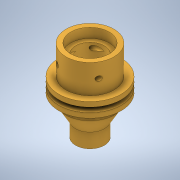
# Autodesk Inventor part: inner element
Saved by Autodesk Inventor 2021 (Build 250183000, 183)
## iProperties
Created: 2021-07-21
Part Number: inner element
Material: Brass, Soft Yellow
Document SubType Name: Modeling
Designer: samlo
Density: 8.47 g/cm^3
Appearance: Brass - Satin
Author: samlo
Autodesk Inventor part; units mm, degrees
ref_plane "YZ Plane" through (0, 0, 0) normal (1, 0, 0) x (0, 1, 0)
ref_plane "XZ Plane" through (0, 0, 0) normal (0, 1, 0) x (-1, 0, 0)
sketch "Sketch1" plane through (0, 0, 0) normal (0, 0, 1) x (1, 0, 0)
  line L0 (2, 0) -> (2, 7)
  line L1 (2, 7) -> (3, 8.7321)
  line L2 (3, 8.7321) -> (3, 15)
  line L3 (3, 15) -> (4, 15)
  line L4 (4, 15) -> (4, 17)
  line L5 (4, 17) -> (5, 17)
  line L6 (5, 17) -> (5, 11)
  line L7 (5, 11) -> (6.5, 11)
  line L8 (6.5, 11) -> (6.5, 10)
  line L9 (6.5, 10) -> (5, 10)
  line L10 (5, 10) -> (5, 9)
  line L11 (5, 9) -> (6.5, 9)
  line L12 (6.5, 9) -> (6.5, 8)
  line L13 (6.5, 8) -> (5, 8)
  line L14 (5, 8) -> (5, 6.4641)
  line L15 (5, 6.4641) -> (3, 3)
  line L16 (3, 3) -> (3, 0)
  line L17 (3, 0) -> (2, 0)
  line L18 (0, -3.4) -> (0, 20.4) projected
  point P0 (0, 0)
  dimension "d0" = 7
  dimension "d1" = 17
  dimension "d2" = 2
  dimension "d3" = 3
  dimension "d4" = 1
  dimension "d5" = 1
  dimension "d6" = 1
  dimension "d7" = 2
  dimension "d8" = 11
  dimension "d9" = 1.5
  dimension "d10" = 5
  dimension "d11" = 60
  dimension "d13" = 4
  dimension "d14" = 3
  dimension "d48" = 4
  constraints: 36 end point, 10 perpendicular, 8 point on line, 2 parallel, 1 vertical
  measures "d0" distance of L0.start L0.end
  measures "d1" vertical distance of L4.end L0.start
  measures "d2" distance of L0.start point (0, 0)
  measures "d3" distance of L16.end point (0, 0)
  measures "d4" distance of L11.end L12.end
  measures "d5" distance of L7.end L8.end
  measures "d6" distance of L9.end L10.end
  measures "d7" distance of L3.end L4.end
  measures "d8" vertical distance of L7.end point (0, 0)
  measures "d9" distance of L12.end L13.end
  measures "d10" horizontal distance of L14.end point (0, 0)
  measures "d11" angle of L17 L1
  measures "d13" distance from line of L4 point (0, 0)
  measures "d14" distance of L15.end L16.end
  measures "d48" distance of L14.end L15.end
revolve "Revolution1" add sketch "Sketch1" angle 360 about axis through (0, -10, 0) along (0, 1, 0)
sketch "Sketch2" plane through (0, 0, 0) normal (1, 0, 0) x (0, 1, 0)
  line L0 (8.7321, 3) -> (15, 3) projected
  point P0 (0, 0)
  point P1 (14, 3)
  dimension "d15" = 1
  dimension "d35" = 3
  constraints: 1 point on line
  measures "d15" distance of L0.end point (14, 3)
  measures "d35" vertical distance of point (0, 0) point (14, 3)
ref_plane "Work Plane1" through (0, 14, 3) normal (0, 0, -1) x (-1, 0, 0)
sketch "Sketch4" plane through (0, 0, 0) normal (1, 0, 0) x (0, 1, 0)
  line L0 (11, 6.5) -> (11, -6.5) projected
  point P0 (0, 0)
  point P1 (14, 2.5)
  dimension "d36" = 3
  dimension "d37" = 2.5
  measures "d36" distance from line of L0 point (14, 2.5)
  measures "d37" vertical distance of point (0, 0) point (14, 2.5)
hole "Hole3" at (0, 14, 2.5) direction (1, 0, 0) diameter 1 end through all
pattern_circular "Circular Pattern2" count 4 over 360 about axis through (0, -10, 0) along (0, 1, 0) of "Hole3"
body "Solid1"
